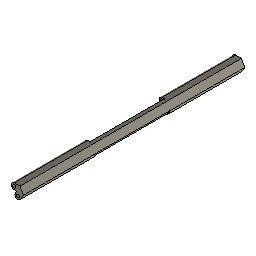
Mothbox_pro_hinge2 (Autodesk Fusion 360 design; units mm, degrees)
Autodesk Fusion 360 part; units mm, degrees
sketch "Sketch1" plane through (0, 0, 0) normal (0, 1, 0) x (1, 0, 0)
  line L0 (0, 0) -> (10, 0)
  line L1 (10, 0) -> (10, -4)
  line L2 (10, -4) -> (0, -4)
  line L3 (0, -4) -> (0, 0)
  circle A0 centre (0, -2) radius 2
  circle A1 centre (10, -2) radius 2
  circle A2 centre (0, -2) radius 1
  circle A3 centre (10, -2) radius 1
  line L4 (5, -4) -> (5, 0)
  circle A4 centre (7.5, -6.3301) radius 1
  circle A5 centre (7.5, -6.3301) radius 2
  line L5 (4.2321, 3.3301) -> (9.2321, -5.3301)
  line L6 (5.7679, -7.3301) -> (0.7679, 1.3301)
  circle A6 centre (2.5, 2.3301) radius 1
  circle A7 centre (2.5, 2.3301) radius 2
  circle A8 centre (7.5, 2.3301) radius 1
  circle A9 centre (7.5, 2.3301) radius 2
  line L7 (0.7679, -5.3301) -> (5.7679, 3.3301)
  line L8 (9.2321, 1.3301) -> (4.2321, -7.3301)
  circle A10 centre (2.5, -6.3301) radius 1
  circle A11 centre (2.5, -6.3301) radius 2
  point P0 (5, -2)
  dimension "d1" = 10
  dimension "d2" = 4
  dimension "d5" = 2
  dimension "d6" = 2
  dimension "d49" = 360
  constraint horizontal L0
  constraint vertical L1
  constraint horizontal L2
  constraint vertical L3
  constraint coincident L0.start L3.end
  constraint midpoint L3 A0.centre
  constraint coincident L0.start A0
  constraint midpoint L1 A1.centre
  constraint coincident L0.end A1
  constraint concentric A0 A2
  constraint concentric A1 A3
  constraint midpoint L2 L4.start
  constraint midpoint L0 L4.end
  constraint midpoint L4 P0
  measures "d1" distance of L0.start L0.end
  measures "d2" distance of L0.start L2.end
  measures "d5" diameter of A2
  measures "d6" diameter of A3
extrude "Extrude1" add sketch "Sketch1" along normal blind 250 contours L3 A0 A2 | L0 L2 A0 L6 L7 | L3 A0 A2 | L0 L5 L6 A7 L7 | L0 L6 L7 | L0 L5 L7 | L0 L2 L4 L6 L7 | L2 L6 L7 | A7 | L0 L2 L4 L5 L8
ref_plane "WorkPlane1" through (0, 51.2, 0) normal (0, 1, 0) x (0, 0, 1)
sketch "Sketch3" plane through (0, 51.2, 0) normal (0, 1, 0) x (1, 0, 0)
  line L0 (-0.4641, -4) -> (-0.4641, 0)
  line L1 (6.1547, -4) -> (0, -4)
  line L2 (0, 0) -> (1.5359, 0)
  line L3 (-0.4641, -4) -> (6.1547, -4)
  line L4 (-0.4641, 0) -> (1.5359, 0)
  circle A0 centre (10, -2) radius 1
  circle A1 centre (10, -2) radius 1
  circle A2 centre (10, -2) radius 2
  arc A3 (10, -4) -> (10, 0) centre (10, -2) ccw
  line L5 (0.7679, 0) -> (3.0774, -4)
  circle A4 centre (-2.116, -8.9952) radius 2
  circle A5 centre (-2.116, -8.9952) radius 1
  line L6 (4.8481, -0.933) -> (1.5387, -6.6651)
  line L7 (4.8481, -0.933) -> (1.384, 1.067)
  line L8 (1.384, 1.067) -> (0.384, -0.6651)
  dimension "d15" = 2
  constraint vertical L0
  constraint coincident L0.start L1
  constraint coincident L0.end L2
  constraint coincident L1.start L3.end
  constraint coincident L2.end L4.end
  constraint equal A0 A1
  constraint concentric A0 A2
  constraint concentric A2 A3
  constraint equal A2 A3
  constraint midpoint L2 L5.start
  constraint midpoint L1 L5.end
  constraint symmetric L0.start L5 L6.start
  constraint symmetric L0.end L5 L7.end
  constraint symmetric L1.start L5 L6.end
  constraint symmetric L2.end L5 L8.end
  constraint symmetric A0 L5 A5
  constraint symmetric A2 L5 A4
  measures "d15" distance of L0.end L2.end
extrude "Extrude3" cut sketch "Sketch3" against normal blind 49.2 contours A2 A3 | A4
ref_plane "WorkPlane2" through (0, 125, 0) normal (0, 1, 0) x (0, 0, 1)
mirror "Mirror1" [no effect]
sketch "Sketch4" plane through (0, 125, 0) normal (0, 1, 0) x (1, 0, 0)
  circle A0 centre (10, -2) radius 1
  circle A1 centre (10, -2) radius 2
  circle A2 centre (0, -2) radius 1
  circle A3 centre (0, -2) radius 2
  circle A4 centre (10, -2) radius 1
  arc A5 (10, -4) -> (10, 0) centre (10, -2) ccw
  arc A6 (0, 0) -> (0, -4) centre (0, -2) ccw
  circle A7 centre (0, -2) radius 1
  line L0 (10, -4) -> (0, -4)
  line L1 (0, 0) -> (10, 0)
  line L2 (5, -4) -> (5, 0)
  line L3 (10, 0) -> (8, 0)
  line L4 (8, 0) -> (8, -4)
  line L5 (2, 0) -> (2, -4)
  circle A8 centre (7.5, -6.3301) radius 1
  circle A9 centre (7.5, -6.3301) radius 2
  line L6 (5.7679, -7.3301) -> (0.7679, 1.3301)
  line L7 (4.2321, 3.3301) -> (9.2321, -5.3301)
  circle A10 centre (2.5, 2.3301) radius 2
  circle A11 centre (2.5, 2.3301) radius 1
  circle A12 centre (7.5, 2.3301) radius 1
  circle A13 centre (7.5, 2.3301) radius 2
  line L8 (9.2321, 1.3301) -> (4.2321, -7.3301)
  line L9 (0.7679, -5.3301) -> (5.7679, 3.3301)
  circle A14 centre (2.5, -6.3301) radius 2
  circle A15 centre (2.5, -6.3301) radius 1
  point P0 (5, -2)
  dimension "d41" = 2
  dimension "d51" = 360
  constraint concentric A0 A1
  constraint concentric A2 A3
  constraint concentric A0 A4
  constraint equal A1 A5
  constraint equal A0 A4
  constraint equal A3 A6
  constraint equal A2 A7
  constraint coincident A5.start L0.start
  constraint coincident A6.end L0.end
  constraint coincident A6.start L1.start
  constraint coincident A5.end L1.end
  constraint midpoint L0 L2.start
  constraint midpoint L1 L2.end
  constraint tangent A5 L3
  constraint coincident L0 L4.end
  constraint perpendicular L0 L4
  constraint symmetric L2 L3.end L5.start
  constraint symmetric L2 L4.end L5.end
  constraint midpoint L2 P0
  measures "d41" distance of A5.end L3.end
extrude "Extrude8" cut sketch "Sketch4" along normal blind 24.6 and the other way blind 24.6 contours L1 L6 L7 A10 L9 | L1 L5 L6 L9 | A10 | L1 L5 L6 | L5 L6 L9 | A3 L1 L5 L6 | A3 L0 L5 L9 | A3 A6
extrude "Extrude5" cut 1 faces at (5, 0, 2) along direction (0, 1, 0) blind 52
extrude "Extrude6" cut 1 faces at (5, 250, 2) along direction (0, -1, 0) blind 52
extrude "Extrude9" cut 1 faces at (6.9245, 149.3333, 2.6667) along direction (-0.866025, 0, -0.5) blind 2 draft 30
fillet "Fillet2" [suppressed]
equation "d7 = 2 mm + 49.2 mm"
